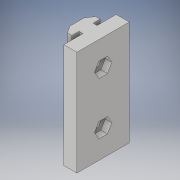
# Autodesk Inventor part: slotMountingPlate_m3Screws
Saved by Autodesk Inventor 2018 (Build 220112000, 112)
## iProperties
Created: 2020-03-14
Part Number: slotMountingPlate_m3Screws
Material: Generic
Document SubType Name: Modeling
Designer: natha
Density: 1 g/cm^3
Appearance: Default
Author: natha
Autodesk Inventor part; units mm, degrees
ref_plane "YZ Plane" through (0, 0, 0) normal (1, 0, 0) x (0, 1, 0)
ref_plane "XZ Plane" through (0, 0, 0) normal (0, 1, 0) x (-1, 0, 0)
ref_plane "XY Plane" through (0, 0, 0) normal (0, 0, 1) x (1, 0, 0)
sketch "Sketch1" plane through (0, 0, 0) normal (0, 1, 0) x (-1, 0, 0)
  line L0 (0, -5.4) -> (1.5, -5.4)
  line L1 (1.5, -5.4) -> (1.5, -8.1)
  line L2 (1.5, -8.1) -> (3.2, -8.1)
  line L3 (0, 0) -> (1.5, 0)
  line L4 (1.5, 0) -> (1.5, 2.7)
  line L5 (1.5, 2.7) -> (3.2, 2.7)
  line L6 (5, 0) -> (5, -5.4)
  line L7 (5, -5.4) -> (3.2, -8.1)
  line L8 (5, 0) -> (3.2, 2.7)
  line L9 (0, -5.4) -> (0, -12.7)
  line L10 (0, -12.7) -> (-5, -12.7)
  line L11 (-5, -12.7) -> (-5, 7.3)
  line L12 (-5, 7.3) -> (0, 7.3)
  line L13 (0, 7.3) -> (0, 0)
  dimension "d0" = 5.4
  dimension "d1" = 1.5
  dimension "d2" = 2.7
  dimension "d3" = 1.7
  dimension "d4" = 2.7
  dimension "d5" = 1.7
  dimension "d9" = 5
  dimension "d10" = 20
  dimension "d11" = 7.3
  constraints: 28 end point, 8 perpendicular, 2 vertical, 1 horizontal, 1 point on line
  measures "d0" distance of L3.start L0.start
  measures "d1" distance of L0.start L0.end
  measures "d2" distance of L0.end L1.end
  measures "d3" distance of L1.end L2.end
  measures "d4" distance of L3.end L4.end
  measures "d5" distance of L4.end L5.end
  measures "d9" distance of L9.end L10.end
  measures "d10" distance between parallel lines of L10 L12
  measures "d11" distance between parallel lines of L3 L12
extrude "Extrusion1" add sketch "Sketch1" along normal blind 40
sketch "Sketch2" plane through (5, 0, 7.3) normal (1, 0, 0) x (0, 0, -1)
  line L0 (11.6599, 7.125) -> (8.3401, 7.125)
  line L1 (8.3401, 7.125) -> (6.6802, 10)
  line L2 (6.6802, 10) -> (8.3401, 12.875)
  line L3 (8.3401, 12.875) -> (11.6599, 12.875)
  line L4 (11.6599, 12.875) -> (13.3198, 10)
  line L5 (13.3198, 10) -> (11.6599, 7.125)
  line L6 (20, 0) -> (0, 0) projected
  line L7 (0, 0) -> (0, 40) projected
  line L8 (11.6599, 27.125) -> (8.3401, 27.125)
  line L9 (8.3401, 27.125) -> (6.6802, 30)
  line L10 (6.6802, 30) -> (8.3401, 32.875)
  line L11 (8.3401, 32.875) -> (11.6599, 32.875)
  line L12 (11.6599, 32.875) -> (13.3198, 30)
  line L13 (13.3198, 30) -> (11.6599, 27.125)
  line L14 (0, 40) -> (20, 40) projected
  point P0 (7.3, 0)
  point P1 (10, 10)
  point P2 (10, 30)
  dimension "d12" = 5.75
  dimension "d13" = 10
  dimension "d14" = 10
  dimension "d15" = 5.75
  dimension "d16" = 10
  dimension "d17" = 10
  constraints: 24 end point, 2 parallel, 26 other
  measures "d12" distance between parallel lines of L3 L0
  measures "d13" distance from line of L6 point (10, 10)
  measures "d14" distance from line of L7 point (10, 10)
  measures "d15" distance between parallel lines of L8 L11
  measures "d16" distance from line of L14 point (10, 30)
  measures "d17" distance from line of L7 point (10, 30)
extrude "Extrusion2" cut sketch "Sketch2" against normal blind 2.5
sketch "Sketch3" plane through (2.5, 0, 7.3) normal (1, 0, 0) x (0, 0, -1)
  point P0 (7.3, 0)
sketch "Sketch4" plane through (2.5, 0, 7.3) normal (1, 0, 0) x (0, 0, -1)
  circle A0 centre (10, 10) radius 1.375
  circle A1 centre (10, 30) radius 1.375
  point P0 (7.3, 0)
  dimension "d20" = 2.75
  dimension "d21" = 2.75
  constraints: 2 centre point
  measures "d20" diameter of A0
  measures "d21" diameter of A1
extrude "Extrusion3" cut sketch "Sketch4" against normal blind 20
body "Solid1"
